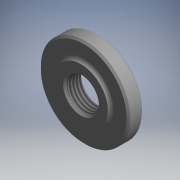
# Autodesk Inventor part: 209407 M8X0,75
Saved by Autodesk Inventor 2021 (Build 250183000, 183)
## iProperties
Part Number: 209407 M8X0,75
Material: Genérico
Catalog Web Link: www.cadenas.de
Description: M8X0,75_R-Raendelmutter
Vendor: FESTO
Document SubType Name: Modeling
Designer: partserver
Manufacturer: FESTO
Mass: 0.965896 g
Surface Area: 8.20361 cm^2
Volume: 0.965896 cm^3
Density: 1 g/cm^3
Appearance: PSOLRGB-175-175-175
Category: PARTsolutions
Company: FESTO
PSOL_IDENT_0: {$CADENAS_DATA\23d-libs\festo\parts\m\msfw\parts\msfw_raendelm.prj},171 {VTYP=3D},{NB=209407 M8X0,75
PSOL_IDENT_1: },{LINA=209407 M8X0,75},{NN=M8X0,75_R},{DATE=09.09.2015 14:47:47},{GEOMDATE=03.09.2015 14:16:04},{VE
PSOL_IDENT_2: RSION=},{LINEID=10},{WBVAR=},{WBNUMERIC=}  {NB=209407 M8X0,75},{LINA=209407 M8X0,75},{KT=DUMMY},{TNR=
PSOL_IDENT_3: 209407},{TYP=M8X0,75}
NB: 209407 M8X0,75
NN: M8X0,75_R
NT: Raendelmutter
NBSYN: $TNR. $TYP.
LINA: 209407 M8X0,75
CATALOG: Festo
TNR: 209407
TYP: M8X0,75
SUPPLIER: FESTO
ARTICLENO: 209407 M8X0,75
BOMINFO: 209407 M8X0,75
CREATOR: CADENAS GmbH
Title: 209407 M8X0,75
Author: Cadenas PARTsolutions
Comments: Raendelmutter
Autodesk Inventor part; units mm, degrees
sketch "Sketch_1" plane through (0, 0, 0) normal (1, 0, 0) x (0, 1, 0)
  line L0 (0, 0) -> (4, 0)
  line L1 (0.406, -3.594) -> (0, -4)
  line L2 (0, -4) -> (0, -6)
  arc A0 (0.6, -6.9165) -> (0, -6) centre (-0.4, -6.9165) ccw
  line L3 (0.6, -6.9165) -> (0.6, -9.6)
  line L4 (0.6, -9.6) -> (1, -10)
  line L5 (1, -10) -> (3.6, -10)
  line L6 (3.6, -10) -> (4, -9.6)
  line L7 (4, -9.6) -> (4, -4)
  line L8 (4, -4) -> (3.594, -3.594)
  line L9 (3.594, -3.594) -> (0.406, -3.594)
  constraints: 20 end point, 2 point on circle, 1 centre point
revolve "Revolution1" add sketch "Sketch_1" angle 360 about axis through (0, 0, 0) along (0, -1, 0)
thread "Thread1" size "M8x0.75" class "6H" standard "ISO Metric profile" full length
ref_plane "ANBAU_XY" through (0, 0, 0) normal (0, 1, 0) x (1, 0, 0)
ref_plane "ANBAU_YZ" through (0, 0, 0) normal (1, 0, 0) x (0, 0, -1)
ref_plane "ANBAU_ZX" through (0, 0, 0) normal (0, 0, -1) x (0, 1, 0)
body "Solid1"
